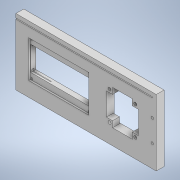
# Autodesk Inventor part: CubeBaseFront
Saved by Autodesk Inventor 2020 (Build 240168000, 168)
## iProperties
Created: 2019-12-01
Part Number: CubeBaseFront
Material: Generic
Document SubType Name: Modeling
Designer: torto
Density: 1 g/cm^3
Appearance: Default
length: 9.000 in
height: 4.250 in
d3: 0.250 in
d4: 0.250 in
d5: 8.750 in
d6: 0.060 in
spacing: 1.417 in
d9: 0.250 in
d10: 0.157 in
d11: 2.000 ul
d13: 1.417 in
thickness: 0.500 in
d19: 0.00 deg
d21: 0.250 in
d22: 0.250 in
d23: 8.750 in
d24: 0.060 in
d25: 0.250 in
d26: 0.00 deg
d33: 0.250 in
d34: 1.417 in
ScrewDiameter: 0.157 in
d36: 0.250 in
d37: 1.417 in
d38: 0.157 in
d39: 2.000 in
d40: 0.00 deg
d49: 2.750 in
d50: 2.125 in
LcdLength: 3.823 in
LcdHeight: 1.567 in
LcdBorderHeight: 2.372 in
LcdBorderLength: 3.868 in
d66: 0.390 in
d67: 0.00 deg
LcdPcbThickness: 0.110 in
d69: 0.00 deg
LcdFrameHoleOffset: 0.098 in
d71: 0.098 in
LcdFrameHoleDiameter: 0.118 in
LcdScrewDepth: 0.236 in
d74: 0.00 deg
InputHeight: 2.245 in
InputLength: 2.050 in
InputThickness: 0.065 in
d78: 0.00 deg
InputHoleSpacing: 0.197 in
d80: 0.197 in
InputScrewDiameter: 0.197 in
d82: 0.394 in
d83: 0.394 in
d84: 0.435 in
d85: 0.00 deg
d86: 0.435 in
d87: 0.00 deg
Author: torto
Autodesk Inventor part; units mm, degrees
ref_plane "YZ Plane" through (0, 0, 0) normal (1, 0, 0) x (0, 1, 0)
ref_plane "XZ Plane" through (0, 0, 0) normal (0, 1, 0) x (-1, 0, 0)
ref_plane "XY Plane" through (0, 0, 0) normal (0, 0, 1) x (1, 0, 0)
sketch "Sketch1" plane through (0, 0, 0) normal (0, 0, 1) x (1, 0, 0)
  line L0 (0, 0) -> (228.6, 0)
  line L1 (228.6, 0) -> (228.6, 107.95)
  line L2 (228.6, 107.95) -> (0, 107.95)
  line L3 (0, 107.95) -> (0, 0)
  line L4 (228.6, 107.95) -> (222.25, 107.95) construction
  line L5 (222.25, 107.95) -> (222.25, 101.6) construction
  line L6 (222.25, 101.6) -> (228.6, 101.6) construction
  line L7 (228.6, 101.6) -> (228.6, 107.95) construction
  line L8 (222.25, 101.6) -> (0, 101.6)
  line L9 (0, 101.6) -> (0, 100.076)
  line L10 (0, 100.076) -> (222.25, 100.076)
  line L11 (222.25, 100.076) -> (222.25, 101.6)
  line L12 (228.6, 0) -> (222.25, 0) construction
  line L13 (222.25, 0) -> (222.25, 35.9833) construction
  line L14 (222.25, 35.9833) -> (228.6, 35.9833) construction
  line L15 (228.6, 35.9833) -> (228.6, 0) construction
  circle A0 centre (222.25, 35.9833) radius 2
  circle A1 centre (222.25, 71.9667) radius 2
  dimension "length" = 228.6
  dimension "height" = 107.95
  dimension "d3" = 6.35
  dimension "d4" = 6.35
  dimension "d5" = 222.25
  dimension "d6" = 1.524
  dimension "spacing" = 35.9833
  dimension "d9" = 6.35
  dimension "d10" = 4
  dimension "d13" = 35.9833
  constraints: 32 end point, 8 parallel, 4 horizontal, 4 perpendicular, 2 centre point, 2 coincident, 1 vertical, 3 other
  measures "length" distance of L2.end L1.end
  measures "height" distance of L1.end L0.end
  measures "d3" distance of L5.end L4.end
  measures "d4" distance of L5.end L6.end
  measures "d5" distance of L10.end L9.end
  measures "d6" distance of L9.end L8.end
  measures "spacing" distance of L12.end L13.end
  measures "d9" distance of L13.end L14.end
  measures "d10" diameter of A0
  measures "d13" distance of A0.centre A1.centre
extrude "Generic Shape" add sketch "Sketch1" along normal blind 12.7
sketch "Sketch2" plane through (0, 0, 12.7) normal (0, 0, 1) x (1, 0, 0)
  line L0 (228.6, 107.95) -> (0, 107.95) construction
  line L1 (228.6, 107.95) -> (222.25, 107.95) construction
  line L2 (222.25, 107.95) -> (222.25, 101.6) construction
  line L3 (222.25, 101.6) -> (228.6, 101.6) construction
  line L4 (228.6, 101.6) -> (228.6, 107.95) construction
  line L5 (222.25, 101.6) -> (0, 101.6)
  line L6 (0, 101.6) -> (0, 100.076)
  line L7 (0, 100.076) -> (222.25, 100.076)
  line L8 (222.25, 100.076) -> (222.25, 101.6)
  point P0 (0, 0)
  dimension "d21" = 6.35
  dimension "d22" = 6.35
  dimension "d23" = 222.25
  dimension "d24" = 1.524
  constraints: 16 end point, 4 parallel, 2 horizontal, 2 perpendicular
  measures "d21" distance of L2.end L1.end
  measures "d22" distance of L2.end L3.end
  measures "d23" distance of L7.end L6.end
  measures "d24" distance of L6.end L5.end
extrude "PCB Notch" cut sketch "Sketch2" against normal blind 6.35
sketch "Sketch4" plane through (0, 0, 0) normal (-1, 0, 0) x (0, 0, 1)
  line L0 (0, 0) -> (6.35, 0) construction
  line L1 (6.35, 0) -> (6.35, 35.9833) construction
  line L2 (6.35, 35.9833) -> (0, 35.9833) construction
  line L3 (0, 35.9833) -> (0, 0) construction
  circle A0 centre (6.35, 35.9833) radius 2
  line L4 (0, 107.95) -> (6.35, 107.95) construction
  line L5 (6.35, 107.95) -> (6.35, 71.9667) construction
  line L6 (6.35, 71.9667) -> (0, 71.9667) construction
  line L7 (0, 71.9667) -> (0, 107.95) construction
  circle A1 centre (6.35, 71.9667) radius 2
  dimension "d33" = 6.35
  dimension "d34" = 35.9833
  dimension "ScrewDiameter" = 4
  dimension "d36" = 6.35
  dimension "d37" = 35.9833
  dimension "d38" = 4
  constraints: 16 end point, 4 parallel, 2 centre point, 2 coincident, 2 horizontal, 2 perpendicular
  measures "d33" distance of L2.end L1.end
  measures "d34" distance of L1.end L0.end
  measures "ScrewDiameter" diameter of A0
  measures "d36" distance of L5.end L6.end
  measures "d37" distance of L4.end L5.end
  measures "d38" diameter of A1
extrude "2in Screw Depth" cut sketch "Sketch4" against normal blind 50.8
sketch "LCD" plane through (0, 0, 0) normal (0, 0, -1) x (-1, 0, 0)
  line L0 (0, 0) -> (-228.6, 0) construction
  line L1 (0, 0) -> (-69.85, 0) construction
  line L2 (-69.85, 0) -> (-69.85, 53.975) construction
  line L3 (-69.85, 53.975) -> (0, 53.975) construction
  line L4 (0, 53.975) -> (0, 0) construction
  line L5 (-118.4, 73.875) -> (-21.3, 73.875)
  line L6 (-21.3, 73.875) -> (-21.3, 34.075)
  line L7 (-21.3, 34.075) -> (-118.4, 34.075)
  line L8 (-118.4, 34.075) -> (-118.4, 73.875)
  line L9 (-118.4, 73.875) -> (-21.3, 34.075) construction
  line L10 (-21.3, 73.875) -> (-118.4, 34.075) construction
  line L11 (-118.975, 84.1) -> (-20.725, 84.1)
  line L12 (-20.725, 84.1) -> (-20.725, 23.85)
  line L13 (-20.725, 23.85) -> (-118.975, 23.85)
  line L14 (-118.975, 23.85) -> (-118.975, 84.1)
  line L15 (-118.975, 84.1) -> (-20.725, 23.85) construction
  line L16 (-20.725, 84.1) -> (-118.975, 23.85) construction
  dimension "d49" = 69.85
  dimension "d50" = 53.975
  dimension "LcdLength" = 97.1
  dimension "LcdHeight" = 39.8
  dimension "LcdBorderHeight" = 60.25
  dimension "LcdBorderLength" = 98.25
  constraints: 32 end point, 6 parallel, 4 midpoint, 3 horizontal, 3 perpendicular
  measures "d49" distance of L2.end L3.end
  measures "d50" distance of L1.end L2.end
  measures "LcdLength" distance of L6.end L7.end
  measures "LcdHeight" distance of L7.end L5.start
  measures "LcdBorderHeight" distance of L11.end L12.end
  measures "LcdBorderLength" distance of L12.end L13.end
extrude "LcdWindow" cut sketch "LCD" against normal blind 9.9 contours L5 L6 L7 L8
sketch "Sketch10" plane through (0, 0, 12.7) normal (0, 0, 1) x (1, 0, 0)
  line L0 (118.975, 84.1) -> (20.725, 84.1) projected
  line L1 (118.975, 23.85) -> (118.975, 84.1) projected
  line L2 (20.725, 23.85) -> (118.975, 23.85) projected
  line L3 (20.725, 84.1) -> (20.725, 23.85) projected
  point P0 (0, 0)
extrude "LcdFrame" cut sketch "Sketch10" against normal blind 2.8
sketch "LcdScrewsSketch" plane through (0, 0, 9.9) normal (0, 0, 1) x (1, 0, 0)
  line L0 (20.725, 23.85) -> (20.725, 84.1) construction
  line L1 (20.725, 84.1) -> (23.225, 84.1) construction
  line L2 (23.225, 84.1) -> (23.225, 81.6) construction
  line L3 (23.225, 81.6) -> (20.725, 81.6) construction
  line L4 (20.725, 81.6) -> (20.725, 84.1) construction
  circle A0 centre (23.225, 81.6) radius 1.5
  line L5 (20.725, 84.1) -> (118.975, 84.1) construction
  line L6 (69.85, 84.1) -> (69.85, 23.85) construction
  line L7 (118.975, 23.85) -> (20.725, 23.85) construction
  line L8 (20.725, 53.975) -> (118.975, 53.975) construction
  line L9 (118.975, 84.1) -> (118.975, 23.85) construction
  circle A1 centre (116.475, 81.6) radius 1.5
  circle A2 centre (23.225, 26.35) radius 1.5
  circle A3 centre (116.475, 26.35) radius 1.5
  point P0 (0, 0)
  dimension "LcdFrameHoleOffset" = 2.5
  dimension "d71" = 2.5
  dimension "LcdFrameHoleDiameter" = 3
  constraints: 12 end point, 4 centre point, 4 midpoint, 3 symmetric about line, 2 parallel, 1 coincident, 1 horizontal, 1 perpendicular, 3 other
  measures "LcdFrameHoleOffset" distance of L2.end L3.end
  measures "d71" distance of L1.end L2.end
  measures "LcdFrameHoleDiameter" diameter of A0
extrude "LcdScrews" cut sketch "LcdScrewsSketch" against normal blind 6
sketch "Sketch12" plane through (0, 0, 0) normal (0, 0, 1) x (1, 0, 0)
  line L0 (118.4, 34.075) -> (118.4, 73.875) construction
  line L1 (118.4, 53.975) -> (228.6, 53.975) construction
  line L2 (228.6, 0) -> (228.6, 107.95) construction
  line L3 (147.465, 82.4865) -> (199.535, 82.4865)
  line L4 (199.535, 82.4865) -> (199.535, 25.4635)
  line L5 (199.535, 25.4635) -> (147.465, 25.4635)
  line L6 (147.465, 25.4635) -> (147.465, 82.4865)
  line L7 (147.465, 82.4865) -> (199.535, 25.4635) construction
  line L8 (199.535, 82.4865) -> (147.465, 25.4635) construction
  point P0 (0, 0)
  point P1 (173.5, 53.975)
  dimension "InputHeight" = 57.023
  dimension "InputLength" = 52.07
  constraints: 14 end point, 5 midpoint, 2 parallel, 1 horizontal, 1 perpendicular
  measures "InputHeight" distance of L5.end L3.start
  measures "InputLength" distance of L4.end L5.end
extrude "InputCountersink" cut sketch "Sketch12" along normal blind 1.66
sketch "Sketch13" plane through (0, 0, 1.66) normal (0, 0, -1) x (-1, 0, 0)
  line L0 (-199.535, 25.4635) -> (-199.535, 82.4865) projected
  line L1 (-199.535, 82.4865) -> (-194.535, 82.4865) construction
  line L2 (-194.535, 82.4865) -> (-194.535, 77.4865) construction
  line L3 (-194.535, 77.4865) -> (-199.535, 77.4865) construction
  line L4 (-199.535, 77.4865) -> (-199.535, 82.4865) construction
  circle A0 centre (-194.535, 77.4865) radius 2.5
  line L5 (-199.535, 82.4865) -> (-147.465, 82.4865) projected
  line L6 (-173.5, 82.4865) -> (-173.5, 25.4635) construction
  line L7 (-147.465, 25.4635) -> (-199.535, 25.4635) projected
  line L8 (-199.535, 53.975) -> (-147.465, 53.975) construction
  line L9 (-147.465, 82.4865) -> (-147.465, 25.4635) projected
  line L10 (-199.535, 82.4865) -> (-189.535, 82.4865) construction
  line L11 (-189.535, 82.4865) -> (-189.535, 72.4865)
  line L12 (-189.535, 72.4865) -> (-199.535, 72.4865)
  line L13 (-199.535, 72.4865) -> (-199.535, 82.4865) construction
  circle A1 centre (-152.465, 77.4865) radius 2.5
  line L14 (-157.465, 82.4865) -> (-157.465, 72.4865)
  line L15 (-157.465, 72.4865) -> (-147.465, 72.4865)
  circle A2 centre (-194.535, 30.4635) radius 2.5
  line L16 (-189.535, 25.4635) -> (-189.535, 35.4635)
  line L17 (-189.535, 35.4635) -> (-199.535, 35.4635)
  circle A3 centre (-152.465, 30.4635) radius 2.5
  line L18 (-157.465, 35.4635) -> (-147.465, 35.4635)
  line L19 (-157.465, 25.4635) -> (-157.465, 35.4635)
  point P0 (0, 0)
  point P1 (-147.465, 35.4635)
  point P2 (-147.465, 72.4865)
  point P3 (-157.465, 82.4865)
  point P4 (-189.535, 25.4635)
  point P5 (-157.465, 25.4635)
  dimension "InputHoleSpacing" = 5
  dimension "d80" = 5
  dimension "InputScrewDiameter" = 5
  dimension "d82" = 10
  dimension "d83" = 10
  constraints: 32 end point, 12 symmetric about line, 4 centre point, 4 midpoint, 4 parallel, 2 horizontal, 2 perpendicular, 1 coincident, 3 other
  measures "InputHoleSpacing" distance of L2.end L3.end
  measures "d80" distance of L1.end L2.end
  measures "InputScrewDiameter" diameter of A0
  measures "d82" distance of L11.end L12.end
  measures "d83" distance of L10.end L11.end
extrude "InputCut" cut sketch "Sketch13" against normal blind 11.04 contours L0 L12 L11 L5 L14 L15 L9 L18 L19 L7 L16 L17
extrude "InputScrews" cut sketch "Sketch13" against normal blind 11.04 contours A0 | A1 | A2 | A3
chamfer "Chamfer1" distance 1.651 angle 45 4 edges at (69.85, 73.875, 0) (118.4, 53.975, 0) (69.85, 34.075, 0) (21.3, 53.975, 0)
equation "\"d3\" = 0.5 * thickness"
equation "\"d4\" = 0.5 * thickness"
equation "\"d5\" = length - 0.5 * thickness"
equation "\"spacing\" = 0.333333 * height"
equation "\"d9\" = 0.5 * thickness"
equation "\"d10\" = ScrewDiameter"
equation "\"d13\" = spacing"
equation "\"d25\" = 0.5 * thickness"
equation "\"d33\" = 0.5 * thickness"
equation "\"d34\" = 0.333333 * height"
equation "\"d36\" = 0.5 * thickness"
equation "\"d37\" = 0.333333 * height"
equation "\"d38\" = ScrewDiameter"
equation "\"d49\" = 0.333333 * length - 0.5 * thickness"
equation "\"d50\" = 0.5 * height"
equation "\"d66\" = thickness - LcdPcbThickness"
equation "\"LcdPcbThickness\" = thickness - LcdThickness"
equation "\"d71\" = LcdFrameHoleOffset"
equation "\"d80\" = InputHoleSpacing"
equation "\"d82\" = 2 * InputHoleSpacing"
equation "\"d83\" = 2 * InputHoleSpacing"
equation "\"d84\" = thickness - InputThickness"
equation "\"d86\" = thickness - InputThickness"
equation "\"LcdThickness\" = 9.9"
equation "\"thickness\" = 12.7"
equation "\"InputThickness\" = 1.66"
body "Solid1"
